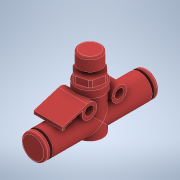
# Autodesk Inventor part: SMC AS2002F Needle Valve RS 827-0755
Saved by Autodesk Inventor 2021 (Build 250183000, 183)
## iProperties
Created: 2020-07-23
Part Number: SMC AS2002F Needle Valve RS 827-0755
Material: Generic
Document SubType Name: Modeling
Designer: jgray
Density: 1 g/cm^3
Appearance: Default
Author: jgray
Autodesk Inventor part; units mm, degrees
ref_plane "YZ Plane" through (0, 0, 0) normal (1, 0, 0) x (0, 1, 0)
ref_plane "XZ Plane" through (0, 0, 0) normal (0, 1, 0) x (-1, 0, 0)
ref_plane "XY Plane" through (0, 0, 0) normal (0, 0, 1) x (1, 0, 0)
sketch "Sketch1" plane through (0, 0, 0) normal (0, 1, 0) x (-1, 0, 0)
  circle A0 centre (0, 0) radius 4.65
  dimension "d0" = 9.3
  constraints: 1 centre point, 1 coincident
  measures "d0" diameter of A0
extrude "Extrusion1" add sketch "Sketch1" along normal blind 14
sketch "Sketch2" plane through (0, 0, 0) normal (1, 0, 0) x (0, 1, 0)
  line L0 (5.1, 19.6063) -> (5.1, -20.5556)
  line L1 (0.45, -18.25) -> (9.75, -18.25)
  line L2 (9.75, -18.25) -> (9.75, 18.25)
  line L3 (9.75, 18.25) -> (0.45, 18.25)
  line L4 (0.45, 18.25) -> (0.45, -18.25)
  line L5 (0.45, -18.25) -> (9.75, 18.25) construction
  line L6 (9.75, -18.25) -> (0.45, 18.25) construction
  point P0 (0, 0)
  point P1 (5.1, 0)
  point P2 (5.1, 18.25)
  point P3 (5.1, -18.25)
  dimension "d3" = 5.1
  dimension "d4" = 9.3
  dimension "d5" = 36.5
  constraints: 14 end point, 2 midpoint, 2 parallel, 1 horizontal, 1 perpendicular, 1 point on line, 1 vertical
  measures "d3" distance from line of point (0, 0) L0
  measures "d4" distance of L3.end L2.end
  measures "d5" distance of L2.end L1.end
revolve "Revolution1" add sketch "Sketch2" angle 360 about axis through (0, 5.1, 19.6063) along (0, 0, -1) contours L3 L2 L1 L0
sketch "Sketch3" plane through (0, 14, 0) normal (0, 1, 0) x (1, 0, 0)
  circle A0 centre (0, 0) radius 5.15
  dimension "d7" = 10.3
  constraints: 1 centre point, 1 coincident
  measures "d7" diameter of A0
extrude "Extrusion2" add sketch "Sketch3" along normal blind 3.2
sketch "Sketch4" plane through (0, 0, 0) normal (1, 0, 0) x (0, 1, 0)
  line L0 (5.1, 29.7602) -> (5.1, -28.3568)
  line L1 (5.1, 0) -> (5.1, 0) projected
  line L2 (5.1, 0) -> (5.1, 0) projected
  line L3 (0.45, 18.25) -> (9.75, 18.25) projected
  line L4 (0.45, -18.25) -> (9.75, -18.25) projected
  line L5 (5.1, 0) -> (5.1, 0) projected
  line L6 (5.1, 0) -> (5.1, 0) projected
  line L7 (5.1, 18.25) -> (7.8, 18.25)
  line L8 (7.8, 18.25) -> (7.8, 19.25)
  line L9 (7.8, 19.25) -> (5.1, 19.25)
  line L10 (5.1, 19.25) -> (5.1, 18.25)
  line L11 (0.45, -18.25) -> (9.75, -18.25) projected
  line L12 (5.1, -18.25) -> (7.8, -18.25)
  line L13 (7.8, -18.25) -> (7.8, -19.25)
  line L14 (7.8, -19.25) -> (5.1, -19.25)
  line L15 (5.1, -19.25) -> (5.1, -18.25)
  line L16 (5.1, 19.25) -> (9.7, 19.25)
  line L17 (9.7, 19.25) -> (9.7, 20.85)
  line L18 (9.7, 20.85) -> (5.1, 20.85)
  line L19 (5.1, 20.85) -> (5.1, 19.25)
  line L20 (5.1, -19.25) -> (9.7, -19.25)
  line L21 (9.7, -19.25) -> (9.7, -20.85)
  line L22 (9.7, -20.85) -> (5.1, -20.85)
  line L23 (5.1, -20.85) -> (5.1, -19.25)
  point P0 (0, 0)
  dimension "d10" = 2.7
  dimension "d11" = 1
  dimension "d12" = 2.7
  dimension "d13" = 1
  dimension "d14" = 4.6
  dimension "d15" = 1.6
  dimension "d16" = 4.6
  dimension "d17" = 1.6
  constraints: 34 end point, 8 parallel, 4 horizontal, 4 perpendicular, 2 midpoint, 1 point on line, 1 vertical
  measures "d10" distance of L9.end L8.end
  measures "d11" distance of L8.end L7.end
  measures "d12" distance of L13.end L14.end
  measures "d13" distance of L12.end L13.end
  measures "d14" distance of L18.end L17.end
  measures "d15" distance of L17.end L16.end
  measures "d16" distance of L21.end L22.end
  measures "d17" distance of L20.end L21.end
revolve "Revolution2" add sketch "Sketch4" angle 360 about axis through (0, 5.1, 29.7602) along (0, 0, -1)
sketch "Sketch5" plane through (0, 0, 0) normal (1, 0, 0) x (0, 1, 0)
  circle A0 centre (11.8, 5.5) radius 1.65
  circle A1 centre (11.8, -5.5) radius 1.65
  arc A2 (13.0912, 7.928) -> (14.4276, 6.3112) centre (11.8, 5.5) ccw
  circle A3 centre (11.8, -5.5) radius 2.75
  line L0 (25.1321, 0) -> (-14.5759, 0)
  line L1 (0, -4.65) -> (0, 4.65) projected
  line L2 (14.4276, 6.3112) -> (11.6216, 15.4)
  line L3 (11.6216, 15.4) -> (10.4522, 15.4)
  line L4 (10.4522, 15.4) -> (10.4522, 14.6)
  line L5 (10.4522, 14.6) -> (11.0313, 14.6)
  line L6 (11.0313, 14.6) -> (13.0912, 7.928)
  point P0 (0, 0)
  dimension "d19" = 3.3
  dimension "d20" = 3.3
  dimension "d21" = 5.5
  dimension "d22" = 5.5
  dimension "d23" = 11.8
  dimension "d24" = 11.8
  dimension "d25" = 5.5
  dimension "d26" = 11
  dimension "d42" = 0.8
  dimension "d43" = 0.8
  dimension "d44" = 15.4
  constraints: 12 end point, 4 centre point, 2 coincident, 2 horizontal, 2 perpendicular, 2 point on circle, 1 parallel, 1 point on line, 1 tangent
  measures "d19" diameter of A0
  measures "d20" diameter of A1
  measures "d21" diameter of A2
  measures "d22" diameter of A3
  measures "d23" distance from line of L1 A1.centre
  measures "d24" distance from line of L1 A0.centre
  measures "d25" distance from line of A0.centre L0
  measures "d26" distance of A1.centre A0.centre
  measures "d42" distance of L3.end L4.end
  measures "d43" distance between parallel lines of L2 L6
  measures "d44" distance between parallel lines of L3 L0
extrude "Extrusion3" add sketch "Sketch5" along normal mid plane 10.6
fillet "Fillet1" radius 0.7 2 edges at (0, 0.5, 20.85) (0, 0.5, -20.85)
fillet "Fillet2" radius 0.7 1 edges at (-5.15, 17.2, 0)
sketch "Sketch6" plane through (0, 17.2, 0) normal (0, 1, 0) x (1, 0, 0)
  line L0 (-4.7915, -0.8985) -> (-3.8633, 2.9733)
  line L1 (-3.1739, 3.7003) -> (0.6433, 4.8324)
  line L2 (1.6176, 4.5988) -> (4.5066, 1.8591)
  line L3 (4.7915, 0.8985) -> (3.8633, -2.9733)
  line L4 (3.1739, -3.7003) -> (-0.6433, -4.8324)
  line L5 (-1.6176, -4.5988) -> (-4.5066, -1.8591)
  circle A0 centre (0, 0) radius 5.15 projected
  arc A1 (-4.7915, -0.8985) -> (-4.5066, -1.8591) centre (0, 0) ccw
  arc A2 (-3.1739, 3.7003) -> (-3.8633, 2.9733) centre (0, 0) ccw
  arc A3 (1.6176, 4.5988) -> (0.6433, 4.8324) centre (0, 0) ccw
  arc A4 (4.7915, 0.8985) -> (4.5066, 1.8591) centre (0, 0) ccw
  arc A5 (-1.6176, -4.5988) -> (-0.6433, -4.8324) centre (0, 0) ccw
  arc A6 (3.1739, -3.7003) -> (3.8633, -2.9733) centre (0, 0) ccw
  dimension "d30" = 8.9
  constraints: 12 end point, 12 point on circle, 6 centre point, 2 coincident, 7 other
  measures "d30" distance between parallel lines of L3 L0
extrude "Extrusion4" add sketch "Sketch6" along normal blind 2.35 contours L0 A2 L1 A3 L2 A4 L3 A6 L4 A5 L5 A1
sketch "Sketch7" plane through (0, 19.55, 0) normal (0, 1, 0) x (1, 0, 0)
  circle A0 centre (0, 0) radius 1.45
  dimension "d35" = 2.9
  constraints: 1 centre point, 1 coincident
  measures "d35" diameter of A0
extrude "Extrusion5" add sketch "Sketch7" along normal blind 2
sketch "Sketch8" plane through (0, 21.55, 0) normal (0, 1, 0) x (1, 0, 0)
  circle A0 centre (0, 0) radius 4
  dimension "d38" = 8
  constraints: 1 centre point, 1 coincident
  measures "d38" diameter of A0
extrude "Extrusion6" add sketch "Sketch8" along normal blind 4.6
fillet "Fillet3" radius 0.7 1 edges at (-4, 26.15, 0)
body "Solid1"
